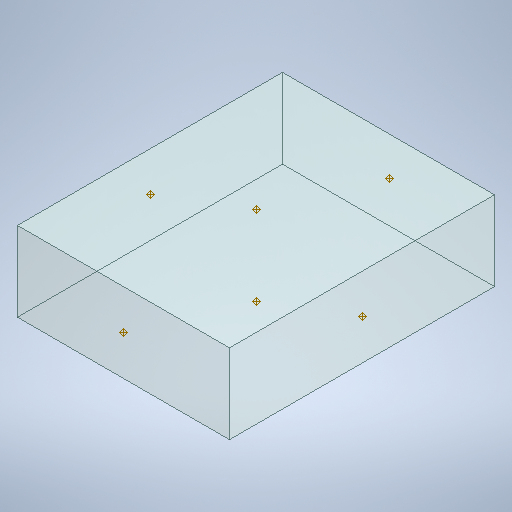
# Autodesk Inventor part: KTN_Chip_4mmX3p2mmX1p2mm
Saved by Autodesk Inventor 2025 (Build 290162000, 162)
## iProperties
Created: 2022-10-12
Part Number: KTN_Chip_4mmX3p2mmX1p2mm
Material: Glass
Document SubType Name: Modeling
Designer: kerlin
Density: 2.18 g/cm^3
Appearance: Clear
Mass: 0.0334848 g
Surface Area: 0.4288 cm^2
Volume: 0.01536 cm^3
Author: kerlin
Autodesk Inventor part; units mm, degrees
ref_plane "YZ Plane" through (0, 0, 0) normal (1, 0, 0) x (0, 1, 0)
ref_plane "XZ Plane" through (0, 0, 0) normal (0, 1, 0) x (-1, 0, 0)
ref_plane "XY Plane" through (0, 0, 0) normal (0, 0, 1) x (1, 0, 0)
sketch "Sketch1" plane through (0, 0, 0) normal (0, 1, 0) x (-1, 0, 0)
  line L0 (1.6, -2) -> (-1.6, -2)
  line L1 (-1.6, -2) -> (-1.6, 2)
  line L2 (-1.6, 2) -> (1.6, 2)
  line L3 (1.6, 2) -> (1.6, -2)
  line L4 (1.6, -2) -> (-1.6, 2) construction
  line L5 (-1.6, -2) -> (1.6, 2) construction
  point P0 (0, 0)
  dimension "d0" = 4
  dimension "d1" = 3.2
  constraints: 12 end point, 2 midpoint, 2 parallel, 1 horizontal, 1 perpendicular
  measures "d0" distance of L0.end L1.end
  measures "d1" distance of L0.start L0.end
extrude "Extrusion1" add sketch "Sketch1" along normal blind 1.2
body "Solid1"
